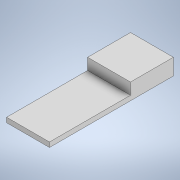
# Autodesk Inventor part: linear_motor_base_upper
Saved by Autodesk Inventor 2022 (Build 260153000, 153)
## iProperties
Created: 2022-08-25
Part Number: linear_motor_base_upper
Material: Generic
Document SubType Name: Modeling
Designer: Alok
Density: 1 g/cm^3
Appearance: Default
Author: Alok
Autodesk Inventor part; units mm, degrees
ref_plane "YZ Plane" through (0, 0, 0) normal (1, 0, 0) x (0, 1, 0)
ref_plane "XZ Plane" through (0, 0, 0) normal (0, 1, 0) x (-1, 0, 0)
ref_plane "XY Plane" through (0, 0, 0) normal (0, 0, 1) x (1, 0, 0)
sketch "Sketch1" plane through (0, 0, 0) normal (0, 1, 0) x (-1, 0, 0)
  line L0 (22.5, 65) -> (-22.5, 65)
  line L1 (-22.5, 65) -> (-22.5, -65)
  line L2 (-22.5, -65) -> (22.5, -65)
  line L3 (22.5, -65) -> (22.5, 65)
  line L4 (22.5, 65) -> (-22.5, -65) construction
  line L5 (-22.5, 65) -> (22.5, -65) construction
  point P0 (0, 0)
  dimension "d0" = 45
  dimension "d1" = 130
  constraints: 12 end point, 2 midpoint, 2 parallel, 1 horizontal, 1 perpendicular
  measures "d0" distance of L2.end L1.end
  measures "d1" distance of L1.end L0.end
extrude "Extrusion1" add sketch "Sketch1" along normal blind 5
sketch "Sketch2" plane through (0, 5, 0) normal (0, 1, 0) x (1, 0, 0)
  line L0 (22.5, 65) -> (-22.5, 65) projected
  line L1 (22.5, -65) -> (22.5, 65) projected
  line L2 (-22.5, 65) -> (22.5, 65)
  line L3 (22.5, 65) -> (22.5, 20)
  line L4 (22.5, 20) -> (-22.5, 20)
  line L5 (-22.5, 20) -> (-22.5, 65)
  point P0 (0, 0)
  dimension "d4" = 45
  constraints: 8 end point, 2 parallel, 1 horizontal, 1 perpendicular, 1 point on line
  measures "d4" distance of L2.end L3.end
extrude "Extrusion2" add sketch "Sketch2" along normal blind 12
body "Solid1"
